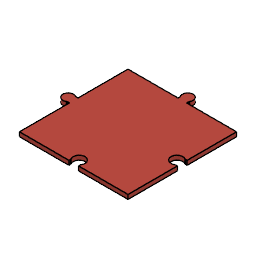
Kidslab Platte (Autodesk Fusion 360 design; units mm, degrees)
Autodesk Fusion 360 part; units mm, degrees
note: some values were not read from the file. Set by a fixed rule: which face or edge a step refers to.
box "Grundkörper Quader1" add length 50 width 50 height 2 placed x (0, 0, 1) y (1, 0, 0) z (0, 1, 0) at (0, 0, 0) makes body 1
sketch "Skizze5" plane through (0, 2, 0) normal (0, 1, 0) x (-1, 0, 0)
  line L0 (0, 50) -> (-50, 50)
  line L1 (-50, 50) -> (-50, 0)
  line L2 (-50, 0) -> (0, 0)
  line L3 (0, 0) -> (0, 50)
  line L4 (-25, 0) -> (-25, 50) construction
  line L5 (-23, 0) -> (-23, -0.6972)
  line L6 (-27, 0) -> (-27, -0.6972)
  arc A0 (-27.1429, -1.2123) -> (-22.8571, -1.2123) centre (-25, -2.5) ccw
  arc A1 (-27.1429, -1.2123) -> (-27, -0.6972) centre (-28, -0.6972) ccw
  arc A2 (-23, -0.6972) -> (-22.8571, -1.2123) centre (-22, -0.6972) ccw
  point P0 (-23, 3)
  dimension "d27" = 5
  dimension "d28" = 2
  dimension "d30" = 3
  constraint midpoint L2 L4.start
  constraint midpoint L0 L4.end
  constraint coincident L2 L5.start
  constraint perpendicular L2 L5
  constraint vertical L4.start A0.centre
  constraint symmetric L4 L5.start L6.start
  constraint tangent L6 A1
  constraint tangent A0 A1
  constraint tangent L5 A2
  constraint tangent A0 A2
  measures "d27" diameter of A0
  measures "d28" distance of L4 L5
  measures "d30" distance of L5.start P0
extrude "Extrusion4" add sketch "Skizze5" against normal blind 2 separate body contours L2 L5 L6 A0 A1 A2 makes body 2
sketch "Skizze7" plane through (0, 2, 0) normal (0, 1, 0) x (-1, 0, 0)
  line L0 (0, 50) -> (-50, 50)
  line L1 (-50, 50) -> (-50, 0)
  line L2 (-50, 0) -> (0, 0)
  line L3 (0, 0) -> (0, 50)
  line L4 (-25, 0) -> (-25, 50) construction
  line L5 (-50, 25) -> (0, 25) construction
  point P0 (-25, 25)
  constraint midpoint L2 L4.start
  constraint midpoint L0 L4.end
  constraint midpoint L1 L5.start
  constraint midpoint L3 L5.end
  constraint midpoint L4 P0
pattern_circular "C-Anordnung1" count 4 over 360 about axis through (25, -48, 25) along (0, 1, 0) of bodies 2 makes body 3 at (-1.4261, 0.6667, 27.2576) makes body 4 at (22.6104, 0.6667, 51.7651) makes body 5 at (51.7651, 0.6667, 27.3896)
mirror "Spiegeln3" about plane through (0, 0, 50) normal (0, 0, 1) of bodies 4 makes body 6
mirror "Spiegeln4" about plane through (50, 0, 0) normal (1, 0, 0) of bodies 5 makes body 7
combine "Kombinieren2" operation add target body 1 tool bodies 3 2
combine "Kombinieren3" operation cut target body 1 tool bodies 6 7
move_face "Flächen versetzen1" offset -0.2 10 faces at (48.2349, 0.6667, 27.3896) (22.6104, 0.6667, 48.2349) (23, 1.3333, 49.7676) (22.8795, 1.3333, 48.8269) (27.001, 1.3333, 49.2577) (27, 1.3333, 49.7676) (49.7676, 1.3333, 23) (48.8269, 0.6667, 22.8795) (49.7676, 1.3333, 27) (49.2577, 0.6667, 27.001) on bodies 1
delete_body "Körper entfernen1" bodies 4
delete_body "Körper entfernen2" bodies 5
equation "d5 = StärkeFläche"
equation "Magnet_Durchmesser = 5 mm"
equation "Magnet_Stärke = 1.5 mm"
equation "Halterung_Breite = 5.5 mm"
equation "StärkeFläche = 2 mm"
equation "d32 = -StärkeFläche"
equation "d40 = Threshold"
equation "Threshold = -0.2 mm"
named bodies: "Platte", "Puzzleteil", "Puzzleteil (1)", "Puzzleteil (2)", "Puzzleteil (3)", "Puzzleteil (2) (1)", "Puzzleteil (3) (1)"
